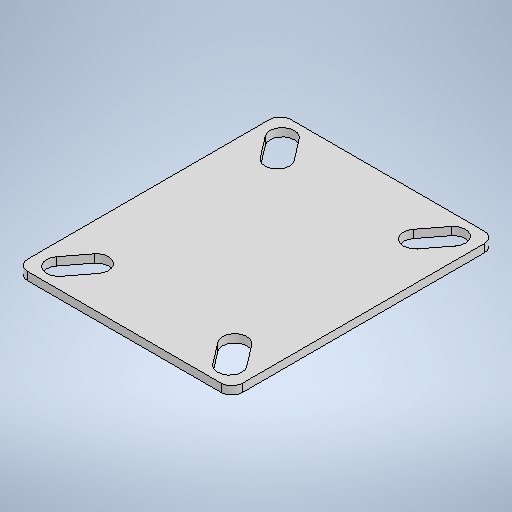
# Autodesk Inventor part: AQUA AISI304 4vv wheel plate 150
Saved by Autodesk Inventor 2025.1 (Build 291241020, 241B)
## iProperties
Created: 2024-11-20
Part Number: AQUA AISI304 4vv wheel plate 150
Material: Stainless Steel
Document SubType Name: Sheet Metal
Designer: user
Mass: 280.619 g
Surface Area: 364.406 cm^2
Volume: 35.0774 cm^3
Density: 8 g/cm^3
Sheet Metal Rule: AISI304 3mm Die 32
Sheet Metal Width: 80.000 mm
Sheet Metal Length: 98.000 mm
Sheet Metal Area: 7840.000 mm^2
Appearance: Default
Flat Pattern Width: 8 cm
Flat Pattern Length: 9.8 cm
Flat Pattern Area: 78.4 cm^2
Author: user
Autodesk Inventor part; units mm, degrees
ref_plane "YZ Plane" through (0, 0, 0) normal (1, 0, 0) x (0, 1, 0)
ref_plane "XZ Plane" through (0, 0, 0) normal (0, 1, 0) x (-1, 0, 0)
ref_plane "XY Plane" through (0, 0, 0) normal (0, 0, 1) x (1, 0, 0)
sketch "Sketch1" plane through (0, 0, 0) normal (0, 0, 1) x (1, 0, 0)
  line L0 (-40, -49) -> (40, -49)
  line L1 (40, -49) -> (40, 49)
  line L2 (40, 49) -> (-40, 49)
  line L3 (-40, 49) -> (-40, -49)
  line L4 (-40, -49) -> (40, 49) construction
  line L5 (40, -49) -> (-40, 49) construction
  point P0 (0, 0)
  dimension "d0" = 80
  dimension "d1" = 98
  measures "d0" distance of L2.end L1.end
  measures "d1" distance of L1.end L0.end
extrude "Plate1" add sketch "Sketch1" along normal blind 3
sketch "Sketch5" plane through (0, 0, 3) normal (0, 0, 1) x (1, 0, 0)
  line L0 (40, -49) -> (-40, -49) construction
  line L1 (40, 49) -> (40, -49) construction
  line L2 (-40, 49) -> (40, 49) construction
  line L3 (-40, -49) -> (-40, 49) construction
  line L4 (40, 49) -> (-40, 49) construction
  line L5 (-31.8479, 41.6146) -> (-25.7704, 33.6733) construction
  line L6 (-35.4215, 38.8797) -> (-29.344, 30.9385)
  line L7 (-22.1968, 36.4082) -> (-28.2744, 44.3495)
  arc A0 (-28.2744, 44.3495) -> (-35.4215, 38.8797) centre (-31.8479, 41.6146) ccw
  arc A1 (-29.344, 30.9385) -> (-22.1968, 36.4082) centre (-25.7704, 33.6733) ccw
  line L8 (0, 0) -> (-37.5, 49) construction
  point P0 (-28.8092, 37.644)
  dimension "d22" = 9
  dimension "d23" = 10
  dimension "d24" = 11
  dimension "d28" = 2.5
  constraints: 10 end point, 4 point on circle, 4 tangent, 2 centre point, 2 point on line, 1 collinear, 1 midpoint, 1 parallel
  measures "d22" diameter of A1
  measures "d23" distance of L5.end L5.start
  measures "d24" distance of L2.start L5.start
  measures "d28" distance of L8.end L2.start
extrude "Cut1" cut sketch "Sketch5" against normal blind 3
mirror "Mirror1" about plane through (0, 0, 0) normal (0, 1, 0) of "Cut1"
mirror "Mirror2" about plane through (0, 0, 0) normal (1, 0, 0) of "Cut1", "Mirror1"
fillet "Corner Round1" radius 4 4 edges at (-40, 49, 1.5) (40, 49, 1.5) (40, -49, 1.5) (-40, -49, 1.5)
equation "\"d25\" = Thickness"
equation "\"d2\" = Thickness"
equation "\"BendReliefWidth\" = Thickness"
equation "\"BendReliefDepth\" = 0.5 * Thickness"
equation "\"CornerReliefSize\" = 4 * Thickness"
equation "\"MinimumRemnant\" = 2 * Thickness"
equation "\"TransitionRadius\" = BendRadius"
equation "\"JacobiRadiusSize\" = BendRadius"
equation "\"GapSize\" = Thickness"
equation "\"Thickness\" = 3"
equation "\"BendRadius\" = 5"
body "Solid1"
